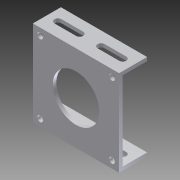
# Autodesk Inventor part: Btm Plate BD Motor mount
Saved by Autodesk Inventor 2012 (Build 160160000, 160)
## iProperties
Created: 2012-06-30
Part Number: Btm Plate BD Motor mount
Material: Default
Document SubType Name: Modeling
Designer: Bruce
Density: 1 g/cm^3
Author: Bruce
Autodesk Inventor part; units mm, degrees
ref_plane "YZ Plane" through (0, 0, 0) normal (1, 0, 0) x (0, 1, 0)
ref_plane "XZ Plane" through (0, 0, 0) normal (0, 1, 0) x (-1, 0, 0)
ref_plane "XY Plane" through (0, 0, 0) normal (0, 0, 1) x (1, 0, 0)
sketch "Sketch1" plane through (0, 0, 0) normal (0, 0, 1) x (1, 0, 0)
  line L0 (-38.1, 38.1) -> (38.1, 38.1)
  line L1 (38.1, 38.1) -> (38.1, -38.1)
  line L2 (38.1, -38.1) -> (-38.1, -38.1)
  line L3 (-38.1, -38.1) -> (-38.1, 38.1)
  circle A0 centre (0, 0) radius 20.5105
  point P0 (-31.75, 31.75)
  point P1 (31.75, 31.75)
  point P2 (31.75, -31.75)
  point P3 (-31.75, -31.75)
  dimension "d0" = 76.2
  dimension "d1" = 76.2
  dimension "d2" = 38.1
  dimension "d3" = 38.1
  dimension "d4" = 41.021
  dimension "d5" = 6.35
  dimension "d6" = 6.35
  dimension "d7" = 6.35
  dimension "d8" = 6.35
  constraints: 8 end point, 2 horizontal alignment, 2 parallel, 2 vertical alignment, 1 centre point, 1 coincident, 1 horizontal, 1 perpendicular
  measures "d0" distance of L2.end L0.start
  measures "d1" distance of L1.end L2.end
  measures "d2" distance from line of L3 point (0, 0)
  measures "d3" distance from line of point (0, 0) L2
  measures "d4" diameter of A0
  measures "d5" distance from line of L0 point (-31.75, 31.75)
  measures "d6" distance from line of L3 point (-31.75, 31.75)
  measures "d7" distance from line of point (31.75, 31.75) L1
  measures "d8" distance from line of L2 point (-31.75, -31.75)
extrude "Extrusion1" add sketch "Sketch1" against normal blind 3.175
hole "Hole1" at (-31.75, 31.75, 0) at (31.75, 31.75, 0) at (31.75, -31.75, 0) at (-31.75, -31.75, 0) direction (0, 0, -1) diameter 5.08 end through all
sketch "Sketch3" plane through (0, 0, -3.175) normal (0, 0, -1) x (-1, 0, 0)
  line L0 (38.1, 38.1) -> (38.1, -38.1) projected
  line L1 (-38.1, -38.1) -> (-38.1, 38.1) projected
  line L2 (38.1, -38.1) -> (-38.1, -38.1) projected
  line L3 (-38.1, 38.1) -> (38.1, 38.1)
  line L4 (38.1, 38.1) -> (38.1, 34.925)
  line L5 (38.1, 34.925) -> (-38.1, 34.925)
  line L6 (-38.1, 34.925) -> (-38.1, 38.1)
  line L7 (-38.1, -34.925) -> (38.1, -34.925)
  line L8 (38.1, -34.925) -> (38.1, -38.1)
  line L9 (38.1, -38.1) -> (-38.1, -38.1)
  line L10 (-38.1, -38.1) -> (-38.1, -34.925)
  dimension "d32" = 3.175
  dimension "d33" = 3.175
  constraints: 16 end point, 4 parallel, 2 horizontal, 2 perpendicular, 2 point on line
  measures "d32" distance between parallel lines of L5 L3
  measures "d33" distance between parallel lines of L2 L7
extrude "Extrusion2" add sketch "Sketch3" along normal blind 21.59 contours L0 L5 L1 L3 | L0 L2 L1 L7
sketch "Sketch4" plane through (-38.1, 38.1, 0) normal (0, 1, 0) x (1, 0, 0)
  line L0 (0, 0) -> (0, 24.765) projected
  line L1 (0, 0) -> (76.2, 0) projected
  line L2 (76.2, 0) -> (76.2, 24.765) projected
  line L3 (6.35, 15.875) -> (31.75, 15.875)
  line L4 (31.75, 15.875) -> (31.75, 9.525)
  line L5 (31.75, 9.525) -> (6.35, 9.525)
  line L6 (6.35, 9.525) -> (6.35, 15.875)
  line L7 (44.45, 15.875) -> (69.85, 15.875)
  line L8 (69.85, 15.875) -> (69.85, 9.525)
  line L9 (69.85, 9.525) -> (44.45, 9.525)
  line L10 (44.45, 9.525) -> (44.45, 15.875)
  point P0 (38.1, 0)
  dimension "d36" = 6.35
  dimension "d37" = 9.525
  dimension "d38" = 6.35
  dimension "d39" = 6.35
  dimension "d40" = 25.4
  dimension "d41" = 6.35
  dimension "d42" = 25.4
  constraints: 16 end point, 4 parallel, 2 horizontal, 2 perpendicular, 1 collinear
  measures "d36" distance of L5.end L3.start
  measures "d37" distance between parallel lines of L1 L5
  measures "d38" distance of L7.end L8.end
  measures "d39" distance between parallel lines of L6 L0
  measures "d40" distance of L3.start L3.end
  measures "d41" distance between parallel lines of L2 L8
  measures "d42" distance of L7.start L7.end
extrude "Extrusion3" cut sketch "Sketch4" against normal through all
fillet "Fillet1" radius 3.175 16 edges at (6.35, 36.5125, -9.525) (6.35, 36.5125, -15.875) (31.75, 36.5125, -15.875) (31.75, 36.5125, -9.525) (-6.35, 36.5125, -9.525) (-6.35, 36.5125, -15.875) (-31.75, 36.5125, -15.875) (-31.75, 36.5125, -9.525) (6.35, -36.5125, -9.525) (6.35, -36.5125, -15.875) (31.75, -36.5125, -15.875) (31.75, -36.5125, -9.525) (-6.35, -36.5125, -9.525) (-6.35, -36.5125, -15.875) (-31.75, -36.5125, -15.875) (-31.75, -36.5125, -9.525)
equation "\"d2\" = 0.5 * d1"
equation "\"d3\" = 0.5 * d0"
equation "\"d7\" = d6"
equation "\"d8\" = d5"
equation "\"d38\" = d36"
equation "\"d41\" = d39"
equation "\"d42\" = d40"
body "Solid1"
